Autodesk Inventor part; units mm, degrees
(part 2 of 2)
  arc A557 (-10.3896, 5.7507) -> (-10.4273, 6.0442) centre (-10.6084, 5.8718) ccw
  arc A558 (-10.3896, 5.7507) -> (-10.4226, 5.6909) centre (0, 0) ccw
  arc A559 (-10.6905, 5.5654) -> (-10.4226, 5.6909) centre (-10.642, 5.8107) ccw
  arc A560 (-11.0673, 5.6599) -> (-10.6905, 5.5654) centre (-9.9441, 9.3385) ccw
  arc A561 (-11.0673, 5.6599) -> (-11.1376, 5.6749) centre (-11.1879, 5.2647) ccw
  arc A562 (-11.1376, 5.6749) -> (-11.6496, 5.7059) centre (-11.6454, 1.5393) ccw
  arc A563 (-11.6496, 5.7059) -> (-11.6946, 5.6778) centre (-11.6496, 5.6559) ccw
  arc A564 (-11.6946, 5.6778) -> (-11.8292, 5.3917) centre (0, 0) ccw
  arc A565 (-11.8292, 5.3917) -> (-11.8223, 5.3391) centre (-11.7837, 5.3709) ccw
  arc A566 (-11.8223, 5.3391) -> (-11.4719, 4.9643) centre (-8.6091, 7.9917) ccw
  arc A567 (-11.4719, 4.9643) -> (-11.4156, 4.9197) centre (-11.188, 5.2646) ccw
  arc A568 (-11.1026, 4.6896) -> (-11.4156, 4.9197) centre (-13.534, 1.7095) ccw
  arc A569 (-11.0285, 4.4032) -> (-11.1026, 4.6896) centre (-11.2607, 4.4959) ccw
  arc A570 (-11.0285, 4.4032) -> (-11.0536, 4.3397) centre (0, 0) ccw
  arc A571 (-11.3037, 4.1817) -> (-11.0536, 4.3397) centre (-11.2863, 4.4311) ccw
  arc A572 (-11.6894, 4.2282) -> (-11.3037, 4.1817) centre (-11.0361, 8.0185) ccw
  arc A573 (-11.6894, 4.2282) -> (-11.761, 4.2342) centre (-11.7596, 3.8209) ccw
  arc A574 (-11.761, 4.2342) -> (-12.2729, 4.2009) centre (-11.7465, 0.0676) ccw
  arc A575 (-12.2729, 4.2009) -> (-12.314, 4.1673) centre (-12.2666, 4.1513) ccw
  arc A576 (-12.314, 4.1673) -> (-12.4117, 3.8666) centre (0, 0) ccw
  arc A577 (-12.4117, 3.8666) -> (-12.3982, 3.8153) centre (-12.3639, 3.8517) ccw
  arc A578 (-12.3982, 3.8153) -> (-12.0037, 3.4874) centre (-9.5428, 6.8497) ccw
  arc A579 (-12.0037, 3.4874) -> (-11.9422, 3.4501) centre (-11.7596, 3.8209) ccw
  arc A580 (-11.6028, 3.2611) -> (-11.9422, 3.4501) centre (-13.6416, -0.0002) ccw
  arc A581 (-11.4934, 2.9863) -> (-11.6028, 3.2611) centre (-11.7353, 3.0491) ccw
  arc A582 (-11.4934, 2.9863) -> (-11.5104, 2.9201) centre (0, 0) ccw
  arc A583 (-11.7387, 2.732) -> (-11.5104, 2.9201) centre (-11.7527, 2.9816) ccw
  arc A584 (-12.1271, 2.7298) -> (-11.7387, 2.732) centre (-11.9541, 6.5721) ccw
  arc A585 (-12.1271, 2.7298) -> (-12.199, 2.7268) centre (-12.1457, 2.3169) ccw
  arc A586 (-12.199, 2.7268) -> (-12.7027, 2.6295) centre (-11.6623, -1.4052) ccw
  arc A587 (-12.7027, 2.6295) -> (-12.7392, 2.5911) centre (-12.6902, 2.5811) ccw
  arc A588 (-12.7392, 2.5911) -> (-12.7984, 2.2805) centre (0, 0) ccw
  arc A589 (-12.7984, 2.2805) -> (-12.7786, 2.2313) centre (-12.7492, 2.2717) ccw
  arc A590 (-12.7786, 2.2313) -> (-12.3461, 1.9554) centre (-10.3261, 5.5997) ccw
  arc A591 (-12.3461, 1.9554) -> (-12.2804, 1.9262) centre (-12.1457, 2.3169) ccw
  arc A592 (-11.9201, 1.7812) -> (-12.2804, 1.9262) centre (-13.534, -1.71) ccw
  arc A593 (-11.777, 1.5222) -> (-11.9201, 1.7812) centre (-12.025, 1.5543) ccw
  arc A594 (-11.777, 1.5222) -> (-11.7856, 1.4544) centre (0, 0) ccw
  arc A595 (-11.9885, 1.2392) -> (-11.7856, 1.4544) centre (-12.0337, 1.485) ccw
  arc A596 (-12.3736, 1.1884) -> (-11.9885, 1.2392) centre (-12.6835, 5.022) ccw
  arc A597 (-12.3736, 1.1884) -> (-12.4445, 1.1764) centre (-12.3403, 0.7764) ccw
  arc A598 (-12.4445, 1.1764) -> (-12.9321, 1.0167) centre (-11.3942, -2.8558) ccw
  arc A599 (-12.9321, 1.0167) -> (-12.9635, 0.974) centre (-12.9136, 0.9703) ccw
  arc A600 (-12.9635, 0.974) -> (-12.9833, 0.6584) centre (0, 0) ccw
  constraints: 1200 point on circle, 601 centre point
extrude "Extrusion1" cut sketch "Sketch_3" along normal blind 3
sketch "Sketch3" plane through (0, 0, 0) normal (0, 0, -1) x (-0.8763067, -0.4817537, 0)
  point P0 (0, 0)
hole "Hole1" at (0, 0, 0) direction (0, 0, 1) diameter 10 depth 3
sketch "_____26" plane through (0, 0, 0) normal (1, 0, 0) x (0, 0, -1)
  line L0 (500, 0) -> (-500, 0)
  line L1 (-0.3, 5) -> (0, 5)
  line L2 (0, 5) -> (0, 5.3)
  line L3 (0, 5.3) -> (-0.3, 5)
  constraints: 8 end point
revolve "Revolution2" cut sketch "_____26" angle 360 about axis through (0, 0, -500) along (0, 0, -1)
sketch "_____27" plane through (0, 0, 0) normal (1, 0, 0) x (0, 0, -1)
  line L0 (500, 0) -> (-500, 0)
  line L1 (-3, 5.3) -> (-3, 5)
  line L2 (-3, 5) -> (-2.7, 5)
  line L3 (-2.7, 5) -> (-3, 5.3)
  constraints: 8 end point
revolve "Revolution3" cut sketch "_____27" angle 360 about axis through (0, 0, -500) along (0, 0, -1)
ref_plane "b_XY" through (0, 0, 0) normal (0, 0, 1) x (1, 0, 0)
ref_plane "b_YZ" through (0, 0, 0) normal (1, 0, 0) x (0, 1, 0)
ref_plane "b_ZX" through (0, 0, 0) normal (0, 1, 0) x (0, 0, 1)
ref_plane "turn_around_XY" through (0, 0, 0) normal (-1, 0, 0) x (0, 0, -1)
ref_plane "turn_around_YZ" through (0, 0, 0) normal (0, 0, -1) x (0, -1, 0)
ref_plane "turn_around_ZX" through (0, 0, 0) normal (0, -1, 0) x (-1, 0, 0)
body "Solid1"
